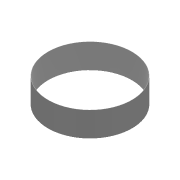
# Autodesk Inventor part: CAR_007_Walls
Saved by Autodesk Inventor 2020 (Build 240168000, 168)
## iProperties
Created: 2020-01-30
Part Number: CAR_007_Walls
Material: Generic
Document SubType Name: Modeling
Designer: user
Density: 1 g/cm^3
Appearance: Polycarbonate - Clear
Mass: 419.364 g
Surface Area: 5336.69 cm^2
Volume: 419.364 cm^3
Author: user
Autodesk Inventor part; units mm, degrees
ref_plane "YZ Plane" through (0, 0, 0) normal (1, 0, 0) x (0, 1, 0)
ref_plane "XZ Plane" through (0, 0, 0) normal (0, 1, 0) x (-1, 0, 0)
ref_plane "XY Plane" through (0, 0, 0) normal (0, 0, 1) x (1, 0, 0)
sketch "Sketch1" plane through (0, 0, 0) normal (0, 1, 0) x (-1, 0, 0)
  circle A0 centre (0, 0) radius 266.7
  circle A1 centre (0, 0) radius 268.2875
  dimension "d1" = 1.5875
  dimension "d4" = 533.4
  constraints: 2 centre point, 1 coincident
  measures "d1" radial gap between concentric circles of A0 A1
  measures "d4" diameter of A0
extrude "Extrusion1" add sketch "Sketch1" along normal blind 157.1752
body "Solid1"
